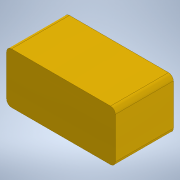
# Autodesk Inventor part: Battery[45x24x21]
Saved by Autodesk Inventor 2020 (Build 240168000, 168)
## iProperties
Created: 2019-12-14
Part Number: Battery[45x24x21]
Material: Polypropylene
Document SubType Name: Modeling
Designer: ermoz
Density: 0.899 g/cm^3
Appearance: Smooth - Ash
Mass: 30.6575 g
Surface Area: 70.8572 cm^2
Volume: 34.1018 cm^3
Author: ermoz
Autodesk Inventor part; units mm, degrees
ref_plane "YZ Plane" through (0, 0, 0) normal (1, 0, 0) x (0, 1, 0)
ref_plane "XZ Plane" through (0, 0, 0) normal (0, 1, 0) x (-1, 0, 0)
ref_plane "XY Plane" through (0, 0, 0) normal (0, 0, 1) x (1, 0, 0)
sketch "Sketch2" plane through (0, 0, 0) normal (0, 1, 0) x (-1, 0, 0)
  line L0 (0, 0) -> (45, 0)
  line L1 (45, 0) -> (45, 24)
  line L2 (45, 24) -> (0, 24)
  line L3 (0, 24) -> (0, 0)
  dimension "d6" = 45
  dimension "d7" = 24
  constraints: 8 end point, 2 parallel, 1 horizontal, 1 perpendicular
  measures "d6" distance of L2.end L1.end
  measures "d7" distance of L1.end L0.end
extrude "Extrusion2" add sketch "Sketch2" along normal blind 21
fillet "Fillet3" radius 2 4 edges at (0, 21, 12) (0, 0, 12) (-45, 21, 12) (-45, 0, 12)
body "Solid2"
